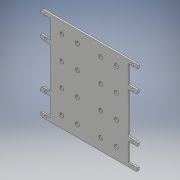
# Autodesk Inventor part: kadlub
Saved by Autodesk Inventor 2018 (Build 220112000, 112)
## iProperties
Created: 2020-10-03
Part Number: kadlub
Material: Ogólny
Document SubType Name: Modeling
Designer: Raven
Density: 1 g/cm^3
Appearance: Domyślna
Author: Raven
Autodesk Inventor part; units mm, degrees
ref_plane "YZ Plane" through (0, 0, 0) normal (1, 0, 0) x (0, 1, 0)
ref_plane "XZ Plane" through (0, 0, 0) normal (0, 1, 0) x (-1, 0, 0)
ref_plane "XY Plane" through (0, 0, 0) normal (0, 0, 1) x (1, 0, 0)
sketch "Szkic1" plane through (0, 0, 0) normal (0, 1, 0) x (-1, 0, 0)
  line L0 (0, 0) -> (50, 0) construction
  line L1 (50, 0) -> (50, -60) construction
  line L2 (50, -60) -> (0, -60) construction
  line L3 (0, -60) -> (0, 0) construction
  line L4 (50, -60) -> (20, -60) construction
  line L5 (20, -60) -> (20, -30) construction
  line L6 (20, -30) -> (50, -30) construction
  line L7 (50, -30) -> (50, -60) construction
  line L8 (20, -30) -> (76.5685, -86.5685) construction
  line L9 (20, -30) -> (100, -30) construction
  line L10 (50, -60) -> (-50, -60)
  line L11 (-50, -60) -> (-50, 60)
  line L12 (-50, 60) -> (50, 60)
  line L13 (50, 60) -> (50, -60)
  dimension "d0" = 50
  dimension "d1" = 60
  dimension "d2" = 30
  dimension "d3" = 30
  dimension "d4" = 80
  dimension "d5" = 45
  dimension "d6" = 100
  dimension "d7" = 120
  constraints: 28 end point, 6 parallel, 4 horizontal, 3 perpendicular, 1 equal length
  measures "d0" distance of L1.end L2.end
  measures "d1" distance of L0.end L1.end
  measures "d2" distance of L5.end L6.end
  measures "d3" distance of L4.end L5.end
  measures "d4" distance of L5.end L8.end
  measures "d5" angle of L8 L9
  measures "d6" distance of L11.end L12.end
  measures "d7" distance of L10.end L11.end
extrude "Wyciągnięcie proste1" add sketch "Szkic1" along normal blind 2
sketch "Szkic2" plane through (0, 0, 0) normal (0, -1, 0) x (1, 0, 0)
  line L0 (-50, 60) -> (-50, -60) construction
  line L1 (50, -60) -> (-50, -60) projected
  line L2 (-50, -60) -> (-62.2, -60)
  line L3 (-62.2, -60) -> (-62.2, -55)
  line L4 (-62.2, -55) -> (-50, -55)
  line L5 (-50, -55) -> (-50, -60)
  line L6 (-56.1, -55) -> (-56.1, -56.9) construction
  circle A0 centre (-56.1, -56.9) radius 1.25
  line L7 (-50, -55) -> (-50, -43.2) construction
  line L8 (-50, -60) -> (-50, 60) construction
  line L9 (-50, -43.2) -> (-68.7012, -43.2) construction
  line L10 (-50, -26.4) -> (-62.2, -26.4)
  line L11 (-62.2, -26.4) -> (-62.2, -31.4)
  line L12 (-62.2, -31.4) -> (-50, -31.4)
  line L13 (-50, -31.4) -> (-50, -26.4)
  line L14 (-56.1, -31.4) -> (-56.1, -29.5) construction
  circle A1 centre (-56.1, -29.5) radius 1.25
  line L15 (0, 0) -> (-82.4094, 0) construction
  line L16 (0, -60) -> (0, 60) construction
  line L17 (-50, -60) -> (-50, 60) construction
  line L18 (50, 60) -> (-50, 60)
  line L19 (-50, 60) -> (-62.2, 60)
  line L20 (-62.2, 60) -> (-62.2, 55)
  line L21 (-62.2, 55) -> (-50, 55)
  line L22 (-50, 55) -> (-50, 60)
  line L23 (-56.1, 55) -> (-56.1, 56.9) construction
  circle A2 centre (-56.1, 56.9) radius 1.25
  line L24 (-50, 55) -> (-50, 43.2) construction
  line L25 (-50, 60) -> (-50, -60) construction
  line L26 (-50, 43.2) -> (-68.7012, 43.2) construction
  line L27 (-62.2, 31.4) -> (-50, 31.4)
  line L28 (-50, 26.4) -> (-62.2, 26.4)
  line L29 (-62.2, 26.4) -> (-62.2, 31.4)
  line L30 (-56.1, 31.4) -> (-56.1, 29.5) construction
  circle A3 centre (-56.1, 29.5) radius 1.25
  line L31 (-50, 31.4) -> (-50, 26.4)
  line L32 (50, 60) -> (50, -60) construction
  line L33 (-50, -60) -> (50, -60)
  line L34 (50, -60) -> (62.2, -60)
  line L35 (62.2, -60) -> (62.2, -55)
  line L36 (62.2, -55) -> (50, -55)
  line L37 (50, -55) -> (50, -60)
  line L38 (56.1, -55) -> (56.1, -56.9) construction
  circle A4 centre (56.1, -56.9) radius 1.25
  line L39 (50, -55) -> (50, -43.2) construction
  line L40 (50, -60) -> (50, 60) construction
  line L41 (50, -43.2) -> (68.7012, -43.2) construction
  line L42 (62.2, -31.4) -> (50, -31.4)
  line L43 (50, -26.4) -> (62.2, -26.4)
  line L44 (62.2, -26.4) -> (62.2, -31.4)
  line L45 (56.1, -31.4) -> (56.1, -29.5) construction
  circle A5 centre (56.1, -29.5) radius 1.25
  line L46 (50, -31.4) -> (50, -26.4)
  line L47 (0, 0) -> (82.4094, 0) construction
  line L48 (62.2, 31.4) -> (50, 31.4)
  line L49 (56.1, 31.4) -> (56.1, 29.5) construction
  circle A6 centre (56.1, 29.5) radius 1.25
  line L50 (62.2, 26.4) -> (62.2, 31.4)
  line L51 (50, 31.4) -> (50, 26.4)
  line L52 (50, 26.4) -> (62.2, 26.4)
  line L53 (50, -60) -> (50, 60) construction
  line L54 (50, 60) -> (50, -60) construction
  line L55 (50, 43.2) -> (68.7012, 43.2) construction
  line L56 (62.2, 55) -> (50, 55)
  line L57 (50, 55) -> (50, 43.2) construction
  line L58 (56.1, 55) -> (56.1, 56.9) construction
  circle A7 centre (56.1, 56.9) radius 1.25
  line L59 (50, 60) -> (62.2, 60)
  line L60 (62.2, 60) -> (62.2, 55)
  line L61 (-50, 60) -> (50, 60)
  line L62 (50, 55) -> (50, 60)
  dimension "d41" = 12.2
  dimension "d42" = 5
  dimension "d43" = 1.9
  dimension "d44" = 2.5
  dimension "d45" = 3.1
  dimension "d46" = 11.8
  constraints: 120 end point, 62 symmetric about line, 8 centre point, 8 coincident, 4 point on line, 2 horizontal, 2 midpoint, 2 parallel, 2 perpendicular, 2 vertical, 7 other
  measures "d41" distance of L3.end L4.end
  measures "d42" distance of L2.end L3.end
  measures "d43" distance of L6.start L6.end
  measures "d44" diameter of A0
  measures "d45" distance from line of L2 L6.end
  measures "d46" distance of L4.end L7.end
extrude "Wyciągnięcie proste2" add sketch "Szkic2" against normal blind 2
sketch "Szkic3" plane through (0, 0, 0) normal (0, -1, 0) x (1, 0, 0)
  circle A0 centre (56.1, -56.9) radius 1.25 construction
  circle A1 centre (56.1, 29.5) radius 1.25 construction
  circle A2 centre (-56.1, 29.5) radius 1.25 construction
  circle A3 centre (-56.1, -56.9) radius 1.25 construction
  circle A4 centre (-56.1, -29.5) radius 1.25 construction
  circle A5 centre (-56.1, 56.9) radius 1.25 construction
  circle A6 centre (56.1, -29.5) radius 1.25 construction
  circle A7 centre (56.1, 56.9) radius 1.25 construction
  line L0 (-62.2, -60) -> (62.2, -60) construction
  line L1 (62.2, -55) -> (62.2, -60) construction
  line L2 (50, -55) -> (62.2, -55) construction
  line L3 (50, -55) -> (50, -31.4) construction
  line L4 (62.2, -31.4) -> (50, -31.4) construction
  line L5 (62.2, -26.4) -> (62.2, -31.4) construction
  line L6 (50, -26.4) -> (62.2, -26.4) construction
  line L7 (50, -26.4) -> (50, 26.4) construction
  line L8 (62.2, 26.4) -> (50, 26.4) construction
  line L9 (62.2, 31.4) -> (62.2, 26.4) construction
  line L10 (50, 31.4) -> (62.2, 31.4) construction
  line L11 (50, 31.4) -> (50, 55) construction
  line L12 (62.2, 55) -> (50, 55) construction
  line L13 (62.2, 60) -> (62.2, 55) construction
  line L14 (62.2, 60) -> (-62.2, 60) construction
  line L15 (-62.2, 60) -> (-62.2, 55) construction
  line L16 (-62.2, 55) -> (-50, 55) construction
  line L17 (-50, 55) -> (-50, 31.4) construction
  line L18 (-50, 31.4) -> (-62.2, 31.4) construction
  line L19 (-62.2, 31.4) -> (-62.2, 26.4) construction
  line L20 (-62.2, 26.4) -> (-50, 26.4) construction
  line L21 (-50, 26.4) -> (-50, -26.4) construction
  line L22 (-50, -26.4) -> (-62.2, -26.4) construction
  line L23 (-62.2, -26.4) -> (-62.2, -31.4) construction
  line L24 (-62.2, -31.4) -> (-50, -31.4) construction
  line L25 (-50, -31.4) -> (-50, -55) construction
  line L26 (-62.2, -55) -> (-50, -55) construction
  line L27 (-62.2, -60) -> (-62.2, -55) construction
  line L28 (-62.2, -60) -> (62.2, -60) construction
  line L29 (62.2, 60) -> (-62.2, 60) construction
  line L30 (-50, 26.4) -> (-50, -26.4) construction
  line L31 (-15, 15) -> (-35, 15) construction
  line L32 (-35, 15) -> (-35, 45) construction
  line L33 (-35, 45) -> (-15, 45) construction
  line L34 (-15, 45) -> (-15, 15) construction
  circle A8 centre (-15, 15) radius 2.5
  circle A9 centre (-35, 15) radius 2.5
  circle A10 centre (-35, 45) radius 2.5
  circle A11 centre (-15, 45) radius 2.5
  line L35 (0, -60) -> (0, 60) construction
  line L36 (50, 0) -> (-50, 0) construction
  line L37 (15, 15) -> (35, 15) construction
  line L38 (35, 15) -> (35, 45) construction
  line L39 (35, 45) -> (15, 45) construction
  line L40 (15, 45) -> (15, 15) construction
  circle A12 centre (15, 15) radius 2.5
  circle A13 centre (35, 15) radius 2.5
  circle A14 centre (35, 45) radius 2.5
  circle A15 centre (15, 45) radius 2.5
  line L41 (-15, -15) -> (-35, -15) construction
  line L42 (-35, -15) -> (-35, -45) construction
  line L43 (-35, -45) -> (-15, -45) construction
  line L44 (-15, -45) -> (-15, -15) construction
  circle A16 centre (-15, -15) radius 2.5
  circle A17 centre (-35, -15) radius 2.5
  circle A18 centre (-35, -45) radius 2.5
  circle A19 centre (-15, -45) radius 2.5
  line L45 (0, 60) -> (0, -60) construction
  line L46 (15, -45) -> (15, -15) construction
  circle A20 centre (15, -45) radius 2.5
  circle A21 centre (15, -15) radius 2.5
  line L47 (35, -45) -> (15, -45) construction
  circle A22 centre (35, -45) radius 2.5
  line L48 (35, -15) -> (35, -45) construction
  line L49 (15, -15) -> (35, -15) construction
  circle A23 centre (35, -15) radius 2.5
  point P0 (0, 0)
  dimension "d52" = 20
  dimension "d53" = 30
  dimension "d54" = 15
  dimension "d55" = 15
  dimension "d56" = 5
  dimension "d57" = 5
  dimension "d58" = 5
  dimension "d59" = 5
  constraints: 38 end point, 26 symmetric about line, 16 centre point, 16 coincident, 4 midpoint, 2 parallel, 1 horizontal, 1 perpendicular, 12 other
  measures "d52" distance of L31.start L31.end
  measures "d53" distance of L31.end L32.end
  measures "d54" distance from line of L21 L31.end
  measures "d55" distance from line of L14 L33.end
  measures "d56" diameter of A8
  measures "d57" diameter of A9
  measures "d58" diameter of A10
  measures "d59" diameter of A11
extrude "Wyciągnięcie proste3" cut sketch "Szkic3" against normal blind 3
fillet "Zaokrąglenie1" radius 2 8 edges at (-62.2, 1, -60) (-62.2, 1, -26.4) (-62.2, 1, 26.4) (-62.2, 1, 60) (62.2, 1, 60) (62.2, 1, 26.4) (62.2, 1, -26.4) (62.2, 1, -60)
fillet "Zaokrąglenie2" radius 2 4 edges at (50, 1, 26.4) (50, 1, -26.4) (-50, 1, -26.4) (-50, 1, 26.4)
equation "\"d57\" = d56"
equation "\"d58\" = d56"
equation "\"d59\" = d56"
